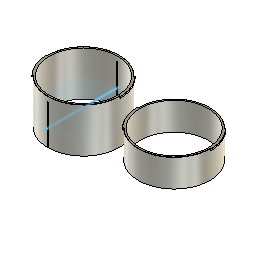
CarHolder_Base_Mount (Autodesk Fusion 360 design; units mm, degrees)
part number: 2025-10-28-13-39-14-687
Autodesk Fusion 360 part; units mm, degrees
sketch "Base late" plane through (0, 0, 0) normal (0, 0, 1) x (1, 0, 0)
  line L0 (-45, 50) -> (45, 50)
  line L1 (50, 45) -> (50, -45)
  line L2 (45, -50) -> (-45, -50)
  line L3 (-50, -45) -> (-50, 45)
  arc A0 (-45, 50) -> (-50, 45) centre (-45, 45) ccw
  arc A1 (50, 45) -> (45, 50) centre (45, 45) ccw
  arc A2 (45, -50) -> (50, -45) centre (45, -45) ccw
  arc A3 (-50, -45) -> (-45, -50) centre (-45, -45) ccw
  point P0 (-50, 50)
  point P1 (50, 50)
  point P2 (-50, -50)
  dimension "d1" = 100
  dimension "d2" = 100
  dimension "d3" = 50
  dimension "d4" = 50
  dimension "d5" = 5
  dimension "d6" = 5
  constraint horizontal L0
  constraint vertical L1
  constraint horizontal L2
  constraint vertical L3
  constraint coincident P0 L0
  constraint coincident P0 L3
  constraint tangent L0 A0
  constraint tangent L3 A0
  constraint coincident P1 L0
  constraint coincident P1 L1
  constraint tangent L0 A1
  constraint tangent L1 A1
  constraint tangent L1 A2
  constraint tangent L2 A2
  constraint equal A1 A2
  constraint coincident P2 L2
  constraint coincident P2 L3
  constraint tangent L2 A3
  constraint tangent L3 A3
  constraint equal A1 A3
  measures "d1" distance of P0 P2
  measures "d2" distance of P0 P1
  measures "d3" distance of origin L0
  measures "d4" distance of origin L3
  measures "d5" radius of A0
  measures "d6" radius of A1
extrude "Extrude1" add sketch "Base late" along normal blind 5 makes body 1
sketch "magnets" plane through (0, 0, 0) normal (0, 0, 1) x (1, 0, 0)
  circle A0 centre (44, -44) radius 5.1
  circle A1 centre (44, 44) radius 5.1
  circle A2 centre (-44, 44) radius 5.1
  circle A3 centre (-44, -44) radius 5.1
  dimension "d32" = 10.2
  dimension "d33" = 10.2
  dimension "d34" = 10.2
  dimension "d35" = 10.2
  measures "d32" diameter of A0
  measures "d33" diameter of A1
  measures "d34" diameter of A2
  measures "d35" diameter of A3
sketch "Extender" plane through (0, 0, 5) normal (0, 0, 1) x (-1, 0, 0)
  arc A0 (45, -50) -> (50, -45) centre (45, -45) ccw
  line L0 (50, -45) -> (50, 45)
  arc A1 (50, 45) -> (45, 50) centre (45, 45) ccw
  line L1 (45, 50) -> (-45, 50)
  arc A2 (-45, 50) -> (-50, 45) centre (-45, 45) ccw
  line L2 (-50, 45) -> (-50, -45)
  arc A3 (-50, -45) -> (-45, -50) centre (-45, -45) ccw
  line L3 (-45, -50) -> (45, -50)
  line L4 (45, -50) -> (37, -50)
  line L5 (37, -50) -> (37, -37)
  line L6 (37, -37) -> (50, -37)
  line L7 (50, -37) -> (50, -45)
  line L8 (-45, -50) -> (-37, -50)
  line L9 (-37, -50) -> (-37, -37)
  line L10 (-37, -37) -> (-50, -37)
  line L11 (-50, -37) -> (-50, -45)
  line L12 (-50, 45) -> (-50, 37)
  line L13 (-50, 37) -> (-37, 37)
  line L14 (-37, 37) -> (-37, 50)
  line L15 (-37, 50) -> (-45, 50)
  line L16 (50, 50) -> (37, 50)
  line L17 (37, 50) -> (37, 37)
  line L18 (37, 37) -> (50, 37)
  line L19 (50, 37) -> (50, 50)
  arc A4 (-45, 50) -> (-50, 45) centre (-45, 45) ccw
  arc A5 (-50, -45) -> (-45, -50) centre (-45, -45) ccw
  arc A6 (45, -50) -> (50, -45) centre (45, -45) ccw
  dimension "d53" = 5
  dimension "d54" = 5
  constraint perpendicular L4 L5
  constraint parallel L4 L6
  constraint parallel L5 L7
  constraint coincident L3 L4.end
  constraint perpendicular L8 L9
  constraint parallel L8 L10
  constraint parallel L9 L11
  constraint coincident L3 L8.end
  constraint perpendicular L12 L13
  constraint parallel L12 L14
  constraint parallel L13 L15
  constraint coincident L2 L12.end
  constraint perpendicular L16 L17
  constraint parallel L16 L18
  constraint parallel L17 L19
  constraint horizontal L16
  constraint tangent L12 A4
  constraint tangent L15 A4
  constraint tangent L8 A5
  constraint tangent L11 A5
  constraint tangent L4 A6
  constraint tangent L7 A6
  constraint equal A5 A6
  measures "d53" radius of A4
  measures "d54" radius of A5
extrude "Extrude10" add sketch "Extender" along normal blind 20 contours A0 L0 L3 L4 L5 L6 L7 A6 | L2 A3 L3 L8 L9 L10 L11 A5 | L0 A1 L1 L16 L17 L18 L19 | L1 A2 L2 L12 L13 L14 L15 A4 bodies 1
sketch "TOP magnets" plane through (0, 0, 25) normal (0, 0, 1) x (-1, 0, 0)
  line L0 (37, -50) -> (45, -50)
  arc A0 (45, -50) -> (50, -45) centre (45, -45) ccw
  line L1 (50, -45) -> (50, -37)
  line L2 (50, -37) -> (37, -37)
  line L3 (37, -37) -> (37, -50)
  circle A1 centre (44, -44) radius 5.1
  circle A2 centre (-44, -44) radius 5.1
  circle A3 centre (-44, 44) radius 5.1
  circle A4 centre (44, 44) radius 5.1
  dimension "d57" = 10.2
  dimension "d58" = 10.2
  dimension "d59" = 10.2
  dimension "d60" = 10.2
  measures "d57" diameter of A1
  measures "d58" diameter of A2
  measures "d59" diameter of A3
  measures "d60" diameter of A4
extrude "Extrude11" cut sketch "TOP magnets" against normal blind 2 contours A1 | A2 | A3 | A4 bodies 1
sketch "Walls" plane through (0, 0, 5) normal (0, 0, 1) x (-1, 0, 0)
  line L0 (37, 37) -> (37, 50)
  line L1 (37, 50) -> (-37, 50)
  line L2 (-37, 50) -> (-37, 37)
  line L3 (-37, 37) -> (-50, 37)
  line L4 (-50, 37) -> (-50, -37)
  line L5 (-50, -37) -> (-37, -37)
  line L6 (-37, -37) -> (-37, -50)
  line L7 (-37, -50) -> (37, -50)
  line L8 (37, -50) -> (37, -37)
  line L9 (37, -37) -> (50, -37)
  line L10 (50, -37) -> (50, 37)
  line L11 (50, 37) -> (37, 37)
  line L12 (37, -50) -> (-37, -50)
  line L13 (-37, -50) -> (-37, -49)
  line L14 (-37, -49) -> (37, -49)
  line L15 (37, -49) -> (37, -50)
  line L16 (-50, -37) -> (-49, -37)
  line L17 (-49, -37) -> (-49, 37)
  line L18 (-49, 37) -> (-50, 37)
  line L19 (-50, 37) -> (-50, -37)
  line L20 (50, -37) -> (49, -37)
  line L21 (49, -37) -> (49, 37)
  line L22 (49, 37) -> (50, 37)
  line L23 (50, 37) -> (50, -37)
  line L24 (37, 50) -> (-37, 50)
  line L25 (-37, 50) -> (-37, 49)
  line L26 (-37, 49) -> (37, 49)
  line L27 (37, 49) -> (37, 50)
  constraint horizontal L12
  constraint vertical L13
  constraint horizontal L14
  constraint vertical L15
  constraint coincident L6 L13.end
  constraint coincident L7.end L8.start
  constraint horizontal L16
  constraint vertical L17
  constraint horizontal L18
  constraint vertical L19
  constraint coincident L3 L17.end
  constraint coincident L4.end L5.start
  constraint horizontal L20
  constraint vertical L21
  constraint horizontal L22
  constraint vertical L23
  constraint coincident L11 L21.end
  constraint coincident L9.end L10.start
  constraint horizontal L24
  constraint vertical L25
  constraint horizontal L26
  constraint vertical L27
  constraint coincident L0.end L1.start
extrude "Extrude12" add sketch "Walls" along normal blind 20 contours L0 L1 L2 L24 L25 L26 L27 | L9 L10 L11 L20 L21 L22 L23 | L3 L4 L5 L16 L17 L18 L19 | L6 L7 L8 L12 L13 L14 L15 bodies 1
hole "Hole2" at (0, 0, 0) direction (0, 0, 1) diameter 85 depth 4 tip angle 180 bodies 1
cylinder "CylinderPrimitive2" cut diameter 87 height 2 placed x (0, 1, 0) y (1, 0, 0) z (0, 0, -1) at (0, 0, 4) bodies 1
sketch "Cutter" plane through (0, 0, 0) normal (0, 0, -1) x (1, 0, 0)
  circle A0 centre (0, 0) radius 42.5
  arc A1 (-50, -45) -> (-45, -50) centre (-45, -45) ccw
  line L0 (-45, -50) -> (45, -50)
  arc A2 (45, -50) -> (50, -45) centre (45, -45) ccw
  line L1 (50, -45) -> (50, 45)
  arc A3 (50, 45) -> (45, 50) centre (45, 45) ccw
  line L2 (45, 50) -> (-45, 50)
  arc A4 (-45, 50) -> (-50, 45) centre (-45, 45) ccw
  line L3 (-50, 45) -> (-50, -45)
  line L4 (0, -50) -> (0, 50)
  line L5 (-50, 0) -> (50, 0)
  line L6 (50, -50) -> (-50, 50)
  line L7 (-50, -50) -> (50, 50)
  arc A5 (30.7591, -30.7591) -> (43.5, 0) centre (0, 0) ccw
  arc A6 (-30.7591, 30.7591) -> (-43.5, 0) centre (0, 0) ccw
  dimension "d84" = 87
  constraint coincident A0.centre A5.centre
  constraint midpoint L0 L4.start
  constraint midpoint L2 L4.end
  constraint midpoint L3 L5.start
  constraint midpoint L1 L5.end
  constraint coincident L6 A5.start
  constraint coincident L5 A6.end
  constraint coincident L6 A6.start
  constraint concentric A5 A6
  constraint coincident L5 A5.end
  measures "d84" diameter of A5
extrude "Extrude14" cut sketch "Cutter" against normal blind 2 contours A0 L5 L6 A5 | A0 L5 L6 A6 bodies 1
cylinder "CylinderPrimitive3" add diameter 86.9 height 30 placed x (0, 1, 0) y (1, 0, 0) z (0, 0, -1) at (0, 0, 4) separate body makes body 2
combine "Combine1" operation cut target body 2 tool bodies 1
sketch "OuterCut" plane through (0, 0, -26) normal (0, 0, -1) x (1, 0, 0)
  circle A0 centre (0, 0) radius 43.45
  circle A1 centre (0, 0) radius 40.5
  dimension "d144" = 81
  constraint concentric A0 A1
  measures "d144" diameter of A1
extrude "Extrude18" cut sketch "OuterCut" against normal blind 30 contours A1 bodies 2
sketch "InnerCut" plane through (0, 0, -26) normal (0, 0, -1) x (1, 0, 0)
  circle A0 centre (0, 0) radius 40.5
  circle A1 centre (0, 0) radius 43.45
  circle A2 centre (0, 0) radius 42.5
  dimension "d147" = 85
  constraint coincident A0.centre A1.centre
  measures "d147" diameter of A2
extrude "Extrude19" cut sketch "InnerCut" against normal blind 26 contours A1 bodies 2
move_face "OffsetFaces1" offset -2.1 1 faces at (41.2921, 3.0944, 4) on bodies 2
fillet "Fillet3" radius 1 2 edges at (-42.975, 0, 1.9) (-42.975, 0, 0) on bodies 2
fillet "Fillet4" radius 1 2 edges at (-30.3879, -30.3879, 1.9) (-30.3879, -30.3879, 0) on bodies 2
fillet "Fillet5" radius 1 2 edges at (42.975, 0, 1.9) (42.975, 0, 0) on bodies 2
fillet "Fillet6" radius 1 2 edges at (30.3879, 30.3879, 0) (30.3879, 30.3879, 1.9) on bodies 2
fillet "Fillet7" radius 0.2 1 edges at (-16.2664, 39.2639, 1.9) on bodies 2
fillet "Fillet8" radius 0.2 1 edges at (16.264, -39.2649, 1.9) on bodies 2
fillet "Fillet9" radius 0.1 3 edges at (-43.449, -0.2929, 1.6071) (-40.1426, -16.6276, 1.9) (-30.9302, -30.516, 1.6071) on bodies 2
fillet "Fillet10" radius 0.1 3 edges at (43.449, 0.2929, 1.6071) (40.1416, 16.6299, 1.9) (30.9509, 30.495, 1.6354) on bodies 2
extrude "Extrude20" add 1 faces at (41.6751, 2.1114, -26) along direction (0, 0, -1) blind 5 on bodies 2 bodies 2
copy_body "CopyPasteBodies1" bodies 2 makes body 3
move_body "Move1" bodies 3 to x (1, 0, 0) y (0, 1, 0) z (0, 0, 1) at (108, 0, 0)
sketch "TorsionCut" plane through (0, 0, -31) normal (0, 0, -1) x (1, 0, 0)
  circle A0 centre (0, 0) radius 42.5
  circle A1 centre (0, 0) radius 40.5
  line L0 (0.25, -43) -> (-0.75, -43)
  line L1 (-0.75, -43) -> (-0.75, 45)
  line L2 (-0.75, 45) -> (0.25, 45)
  line L3 (0.25, 45) -> (0.25, -43)
  dimension "d172" = 1
  dimension "d173" = 88
  constraint horizontal L0
  constraint vertical L1
  constraint horizontal L2
  constraint vertical L3
  measures "d172" distance of L1.end L2.end
  measures "d173" distance of L0.end L1.end
extrude "Extrude22" cut sketch "TorsionCut" against normal blind 27 contours A0 A1 L1 L3 | A0 L1 L2 L3 | A0 L0 L1 L3 | A0 A1 L1 L3 | A1 L1 L3 bodies 2
extrude "Extrude23" add sketch "TorsionCut" along normal blind 20 contours A0 A1 L3 | A0 A1 L1 bodies 2
named bodies: "CarHolderHome", "Mount", "Mount (1)"
